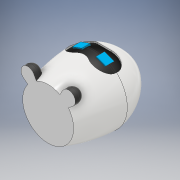
# Autodesk Inventor part: learnbot3
Saved by Autodesk Inventor 2017 (Build 210142000, 142)
## iProperties
Part Number: learnbot3
Material: Genérico
Document SubType Name: Modeling
Designer: rober
Density: 1 g/cm^3
Appearance: Valor por defecto
Author: rober
Autodesk Inventor part; units mm, degrees
ref_plane "YZ Plane" through (0, 0, 0) normal (1, 0, 0) x (0, 1, 0)
sketch "Boceto7" plane through (0, 0, 0) normal (0, 0, 1) x (1, 0, 0)
  line L0 (0, 0) -> (-3, 0)
  arc A0 (-0.8701, 9.6654) -> (-4, 5.3245) centre (1.576, 4.6029) ccw
  arc A1 (-4, 5.3245) -> (-3, 0) centre (13.4839, 5.852) ccw
  arc A2 (0, 9.8646) -> (-0.8701, 9.6654) centre (0, 7.8646) ccw
  line L1 (0, 0.3) -> (-2.7868, 0.3)
  arc A3 (-3.6994, 5.3094) -> (-2.7868, 0.3) centre (13.4839, 5.852) ccw
  arc A4 (-0.7396, 9.3953) -> (-3.6994, 5.3094) centre (1.576, 4.6029) ccw
  arc A5 (0, 9.5646) -> (-0.7396, 9.3953) centre (0, 7.8646) ccw
  line L2 (0, 0) -> (0, 0.3)
  line L3 (0, 9.5646) -> (0, 9.8646)
  dimension "d25" = 0.3
  constraints: 12 point on circle, 8 end point, 6 centre point, 1 collinear, 1 tangent, 1 vertical, 3 other
  measures "d25" radial gap between concentric circles of A0 A4
revolve "Revolución2" add sketch "Boceto7" angle 360 about axis through (0, 9.5646, 0) along (0, 1, 0)
ref_plane "Plano de trabajo2" through (0, 0, 5) normal (0, 0, 1) x (1, 0, 0)
sketch "Boceto10" plane through (0, 0, 5) normal (0, 0, 1) x (1, 0, 0)
  line L0 (0, 0) -> (0, -4.067)
  arc A0 (0.8186, 4.0244) -> (-0.8186, 4.0244) centre (0, 2.6512) ccw
  arc A1 (-0.8186, 6.6245) -> (0.8277, 6.6281) centre (-0.0001, 8.7418) ccw
  arc A2 (0.6088, 4.1295) -> (0.8277, 6.6281) centre (1.3382, 5.3245) ccw
  arc A3 (-0.8186, 6.6245) -> (-0.6088, 4.1295) centre (-1.3382, 5.3245) ccw
  point P0 (-4, 5.3245)
  point P1 (-4, 5.3245)
  constraints: 12 point on circle, 4 centre point, 2 end point, 1 symmetric about line, 1 vertical
extrude "Extrusión4" cut sketch "Boceto10" against normal blind 3 contours A0 A3 A1 A2
sketch "Boceto11" plane through (0, 0, 0) normal (0, 1, 0) x (-1, 0, 0)
  line L0 (0.7384, -5.6858) -> (0.7384, -3.8715) projected
  circle A0 centre (0, 0) radius 3 projected
  line L1 (2.1933, 1.661) -> (2.8944, 2.2113)
  line L2 (1.3218, 2.5458) -> (1.7049, 3.2296)
  arc A1 (1.3218, 2.5458) -> (2.3653, 1.796) centre (1.8859, 2.2298) ccw
  arc A2 (2.8944, 2.2113) -> (1.7049, 3.2296) centre (2.4014, 2.8393) ccw
  line L3 (0, 0) -> (0, -2.3597)
  arc A3 (-2.3653, 1.796) -> (-1.3218, 2.5458) centre (-1.8859, 2.2298) ccw
  line L4 (-1.3218, 2.5458) -> (-1.7049, 3.2296)
  arc A4 (-1.7049, 3.2296) -> (-2.8944, 2.2113) centre (-2.4014, 2.8393) ccw
  line L5 (-2.1933, 1.661) -> (-2.8944, 2.2113)
  point P0 (0, 0)
  constraints: 10 end point, 10 point on circle, 7 symmetric about line, 4 centre point, 3 tangent, 2 point on line, 1 vertical, 2 other
extrude "Extrusión5" add sketch "Boceto11" along normal blind 1.2 contours L1 A1 L2 A0 | A0 L2 A2 L1 | L5 A4 L4 A0 | A0 L4 A3 L5
fillet "Empalme1" radius 0.73 3 edges at (-2.9206, 1.2, 3.4458) (-1.638, 1.2, 3.11) (-2.7904, 1.2, 2.1297)
fillet "Empalme2" radius 0.73 3 edges at (2.9206, 1.2, 3.4458) (2.7904, 1.2, 2.1297) (1.638, 1.2, 3.11)
sketch "Boceto12" plane through (0, 0, 0) normal (1, 0, 0) x (0, 1, 0)
  arc A0 (5.3094, -3.6994) -> (9.3953, -0.7396) centre (4.6029, 1.576) ccw projected
  arc A1 (0.3, -2.7868) -> (5.3094, -3.6994) centre (5.852, 13.4839) ccw projected
  arc A2 (5.3094, -3.6994) -> (9.3953, -0.7396) centre (4.6029, 1.576) ccw projected
  line L0 (0, 0) -> (11.5313, 0)
  arc A3 (7.572, 2.8414) -> (5.4063, 3.6855) centre (4.6029, -1.576) ccw
  arc A4 (7.572, 2.8414) -> (5.3094, 3.6994) centre (4.6029, -1.576) ccw
  arc A5 (5.4063, 3.6855) -> (5.2185, 3.6963) centre (5.2554, 2.697) ccw
  arc A6 (5.4054, 3.8371) -> (5.213, 3.8462) centre (5.2554, 2.697) ccw
  arc A7 (7.6718, 2.9548) -> (5.4054, 3.8371) centre (4.6029, -1.576) ccw
  line L1 (5.3824, 3.8399) -> (5.3828, 3.8406)
  line L2 (0.3, 2.7868) -> (0.3, 2.9452)
  line L3 (0.47, 2.7997) -> (0.47, 3.2296) projected
  line L4 (9.3953, 0.7396) -> (9.5408, 0.7827)
  line L5 (5.3094, 3.8457) -> (5.3094, 3.6994)
  line L6 (5.4054, 3.8371) -> (5.3094, 3.6994)
  line L7 (7.572, 2.8414) -> (7.6718, 2.9548)
  line L8 (2.965, 3.4638) -> (2.9551, 3.6143)
  arc A8 (5.213, 3.8462) -> (2.9551, 3.6143) centre (5.852, -13.4839) ccw
  arc A9 (0.47, 3.0017) -> (0.3, 2.9452) centre (5.852, -13.4839) ccw
  arc A10 (5.2185, 3.6963) -> (2.965, 3.4638) centre (5.852, -13.4839) ccw
  arc A11 (0.47, 2.8438) -> (0.3, 2.7868) centre (5.852, -13.4839) ccw
  arc A12 (7.572, 2.8414) -> (5.3094, 3.6994) centre (4.6029, -1.576) ccw
  point P0 (2.7784, 3.5834)
  point P1 (2.1102, 3.2958)
  dimension "d40" = 1
  dimension "d41" = 0.15
  constraints: 22 point on circle, 16 end point, 10 centre point, 7 symmetric about line, 2 point on line, 1 horizontal, 1 parallel, 1 tangent, 1 vertical, 2 other
  measures "d40" radius of A5
  measures "d41" radial gap between concentric circles of A5 A6
revolve "Revolución3" add sketch "Boceto12" angle 90 mid plane about axis through (0, 0, 0) along (0, 1, 0) contours A3 A4 L6 A7 L7 | A5 A10 L8 A8 A6 L5 A4 | L5 A6 L6
ref_plane "Plano de trabajo3" through (0, 5.3, 0) normal (0, 1, 0) x (-1, 0, 0)
sketch "Boceto13" plane through (0, 5.3, 0) normal (0, 1, 0) x (-1, 0, 0)
  arc A0 (2.7197, 2.7197) -> (-2.7197, 2.7197) centre (0, 0) ccw projected
  line L0 (0, 2.0985) -> (-2.4704, 4.7031)
  line L1 (0, 0) -> (0, -1.7998)
  line L2 (1.8357, 3.3073) -> (0.7716, 3.6925)
  line L3 (0.7716, 3.6925) -> (0.837, 3.8731)
  line L4 (0.837, 3.8731) -> (1.9849, 3.4576)
  line L5 (1.9849, 3.4576) -> (1.8357, 3.3073)
  arc A1 (2.7197, 2.7197) -> (-2.7197, 2.7197) centre (0, 0) ccw
  line L6 (-1.8357, 3.3073) -> (-0.7716, 3.6925)
  line L7 (-0.7716, 3.6925) -> (-0.837, 3.8731)
  line L8 (-0.837, 3.8731) -> (-1.9849, 3.4576)
  line L9 (-1.9849, 3.4576) -> (-1.8357, 3.3073)
  constraints: 20 end point, 6 symmetric about line, 2 perpendicular, 2 point on circle, 1 centre point, 1 vertical, 1 other
extrude "Extrusión6" add sketch "Boceto13" along normal mid plane 1
